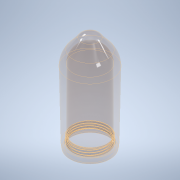
# Autodesk Inventor part: Lumipositor2-Top-V1
Saved by Autodesk Inventor 2022 (Build 260153000, 153)
## iProperties
Created: 2021-10-27
Part Number: Lumipositor2-Top-V1
Material: PC/ABS Plastic
Document SubType Name: Modeling
Designer: incep
Density: 0.357273 g/cm^3
Appearance: Polycarbonate - Smoked
Author: incep
## iProperties of the stored document Lumipositor2-Top-V1_3DPrint.ipt
Created: 2021-10-28
Part Number: Lumipositor2-Top-V1_3DPrint
Material: Generic
Document SubType Name: Modeling
Designer: incep
Density: 1 g/cm^3
Appearance: Default
Author: incep
Autodesk Inventor part; units mm, degrees
ref_plane "YZ Plane" through (0, 0, 0) normal (1, 0, 0) x (0, 1, 0)
ref_plane "XZ Plane" through (0, 0, 0) normal (0, 1, 0) x (-1, 0, 0)
ref_plane "XY Plane" through (0, 0, 0) normal (0, 0, 1) x (1, 0, 0)
sketch "Sketch1" plane through (0, 0, 0) normal (0, 0, 1) x (1, 0, 0)
  circle A0 centre (0, -5) radius 18.5 construction
  line L0 (16.5, -10) -> (17.8115, -10)
  circle A1 centre (0, 53) radius 20 construction
  circle A2 centre (0, 69) radius 10 construction
  line L1 (0, 0) -> (0, 97.7012) construction
  line L2 (-35, 70) -> (35, 70) construction
  line L3 (18.5, -5) -> (19.6723, 53)
  line L4 (7.8062, 75.25) -> (15.2889, 65.9042)
  line L5 (0, 79) -> (0, 70)
  line L6 (15, 55) -> (15, 0)
  arc A3 (19.6723, 53) -> (15.2889, 65.9042) centre (-0.3236, 53.4042) ccw
  arc A4 (17.8115, -10) -> (18.5, -5) centre (0, -5) ccw
  line L7 (16.5, -10) -> (16.5, -6.2)
  line L8 (16.5, -6.2) -> (15.5, -6.2)
  line L9 (15.5, -6.2) -> (15.5, -1.8404)
  line L10 (15.5, -1.8404) -> (15.5, 0)
  line L11 (15.5, 0) -> (15, 0)
  circle A5 centre (0, 55) radius 15 construction
  arc A6 (15, 55) -> (0, 70) centre (0, 55) ccw
  arc A7 (7.8062, 75.25) -> (0, 79) centre (0, 69) ccw
  arc A8 (-9.2846, 70.7143) -> (-9.3884, 70) centre (0, 69) ccw
  point P0 (0, -10)
  point P1 (15, -10)
  dimension "d6" = 20
  dimension "d113" = 40
  dimension "d0" = 5
  dimension "d1" = 5
  dimension "d2" = 37
  dimension "d8" = 70
  dimension "d10" = 70
  dimension "d12" = 3.8
  dimension "d13" = 16.5
  dimension "d14" = 15.5
  dimension "d114" = 15
  dimension "d115" = 30
  dimension "d116" = 16
  dimension "d117" = 2
  constraints: 24 end point, 10 point on circle, 7 centre point, 6 point on line, 5 vertical alignment, 3 coincident, 3 perpendicular, 3 tangent, 2 concentric, 2 horizontal, 2 horizontal alignment, 2 vertical, 1 collinear, 1 midpoint, 9 other
  measures "d0" distance of L1.start A0.centre
  measures "d1" distance from line of L0 A0.centre
  measures "d2" diameter of A0
  measures "d8" distance of L5.end L1.start
  measures "d10" distance of L2.start L2.end
  measures "d12" distance of L0.start L7.end
  measures "d13" distance from line of L7 point (0, -10)
  measures "d14" distance from line of L9 point (0, -10)
  measures "d114" distance from line of L6 L1.start
  measures "d115" diameter of A5
  measures "d116" distance of point (0, 69) point (0, 53)
  measures "d117" distance of point (0, 53) A5.centre
revolve "Revolution1" add sketch "Sketch1" angle 360 about axis through (0, 0, 0) along (0, 1, 0)
thread "Thread4" size "M32x2" class "6H" standard "ANSI Metric M Profile" length 6.2
sketch "Sketch11" plane through (0, -6.2, 0) normal (-1, 0, 0) x (0, 0, 1)
  line L0 (15.5, 0) -> (15.5, 6.2)
  line L1 (15.5, 6.2) -> (14.0171, 6.2)
  line L2 (14.0171, 6.2) -> (14.0171, 0)
  line L3 (14.0171, 0) -> (15.5, 0)
  line L4 (0, -1.24) -> (0, 7.44) projected
  constraints: 8 end point
revolve "Revolution6" add sketch "Sketch11" angle 360 about axis through (0, -6.2, 0) along (0, 1, 0) separate body
sketch "Sketch10" plane through (0, -6.2, 15.5) normal (1, 0, 0) x (0, 1, 0)
  line L0 (-1.1668, -0.1013) -> (-1.0001, -0.1013) construction
  line L1 (0.1666, -1.382) -> (-0.0001, -1.7021) construction
  line L2 (-2.0001, -1.7021) -> (-2.1668, -1.382) construction
  line L3 (-0.8334, -0.1013) -> (-1.0001, 0.2189) construction
  line L4 (-1.0001, 0.2189) -> (-1.1668, -0.1013) construction
  line L5 (-2.0001, -1.7021) -> (-1.8334, -1.382) construction
  line L6 (-0.8334, -0.1013) -> (-0.1668, -1.382)
  line L7 (-2.1668, -1.382) -> (-1.8334, -1.382) construction
  arc A0 (-2.1668, -1.382) -> (-2.0001, -1.4831) centre (-2.0001, -1.2952) ccw construction
  line L8 (0.1666, -1.382) -> (-0.1668, -1.382) construction
  line L9 (-2.0001, -1.7021) -> (-2.0001, -1.382) construction
  line L10 (-0.0001, -1.7021) -> (-0.0001, -1.382) construction
  line L11 (-1.0001, 0.2189) -> (-1.0001, -0.0002) construction
  line L12 (-2.0001, -1.4831) -> (-0.0001, -1.4831)
  arc A1 (-2.0001, -1.4831) -> (-1.8334, -1.382) centre (-2.0001, -1.2952) ccw
  line L13 (-0.1668, -1.382) -> (-0.0001, -1.7021) construction
  line L14 (-1.8334, -1.382) -> (-1.1668, -0.1013)
  line L15 (-0.0001, -0.0002) -> (-0.0001, 0.0177)
  line L16 (-0.0001, 0.0177) -> (-0.0001, -0.0002)
  line L17 (-0.0001, -0.0002) -> (0.0334, -0.0002)
  arc A2 (-0.1668, -1.382) -> (-0.0001, -1.4831) centre (-0.0001, -1.2952) ccw
  arc A3 (-0.0001, -1.4831) -> (0.1666, -1.382) centre (-0.0001, -1.2952) ccw construction
  arc A4 (-1.0001, -0.0002) -> (-1.1668, -0.1013) centre (-1.0001, -0.1881) ccw
  arc A5 (-0.8334, -0.1013) -> (-1.0001, -0.0002) centre (-1.0001, -0.1881) ccw
  line L18 (-1.0001, -0.0002) -> (-1.0001, -0.1013) construction
  line L19 (-1.0001, -0.1013) -> (-0.8334, -0.1013) construction
  dimension "d95" = 55
  dimension "d96" = 0.3202
  dimension "d97" = 0.3202
  dimension "Sketch10_ThreadOffset" = 0
  dimension "Sketch10_MajorRadius" = 1.4829
  dimension "d100" = 2
  dimension "Sketch10_MinorRadius" = 0
  constraints: 40 end point, 12 point on circle, 10 parallel, 8 tangent, 6 centre point, 6 collinear, 2 midpoint, 2 point on line, 1 horizontal, 1 perpendicular, 3 other
  measures "d95" angle of L6 L14
  measures "d96" distance of L3.end L0.end
  measures "d97" distance of L1.end L10.end
  measures "Sketch10_ThreadOffset" distance between parallel lines of L15 L10
  measures "Sketch10_MajorRadius" distance from line of L12 L15.start
  measures "d100" distance from line of L1.end L9
  measures "Sketch10_MinorRadius" distance edge to line of A5 L17
coil "Coil5" sketch "Sketch10" operation cut axis through (0, -6.2, 0) along (0, 1, 0) pitch 2.002 turns 5.094905 hand right bodies 2
equation "\"d95\" = d102"
equation "\"d96\" = 0.160083 * Sketch10_Pitch"
equation "\"d97\" = 0.160083 * Sketch10_Pitch"
equation "\"d100\" = Sketch10_Pitch"
equation "\"d24\" = 55deg"
equation "\"Sketch2_Pitch\" = 2"
equation "\"d44\" = 55deg"
equation "\"Sketch4_Pitch\" = 3.5"
equation "\"d62\" = 55deg"
equation "\"Sketch6_Pitch\" = 2"
equation "\"d82\" = 55deg"
equation "\"Sketch8_Pitch\" = 2"
equation "\"d102\" = 55deg"
equation "\"Sketch10_Pitch\" = 2"
body "Solid1"
body "Solid6"
